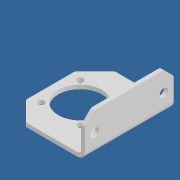
# Autodesk Inventor part: Belt_Unit_Motor_Holder
Saved by Autodesk Inventor 2020 (Build 240168000, 168)
## iProperties
Created: 2021-05-12
Part Number: Belt_Unit_Motor_Holder
Material: 一般
Document SubType Name: Sheet Metal
Designer: ken113
Density: 1 g/cm^3
Sheet Metal Rule: Default_mm
Appearance: 既定
Author: ken113
Autodesk Inventor part; units mm, degrees
ref_plane "YZ Plane" through (0, 0, 0) normal (1, 0, 0) x (0, 1, 0)
ref_plane "XZ Plane" through (0, 0, 0) normal (0, 1, 0) x (-1, 0, 0)
ref_plane "XY Plane" through (0, 0, 0) normal (0, 0, 1) x (1, 0, 0)
sketch "スケッチ1" plane through (0, 0, 0) normal (0, 1, 0) x (-1, 0, 0)
  line L0 (0, -22.5) -> (40, -22.5)
  line L1 (40, -22.5) -> (40, 22.5)
  line L2 (40, 22.5) -> (0, 22.5)
  line L3 (0, 22.5) -> (0, -22.5)
  point P0 (0, 0)
  dimension "d0" = 40
  dimension "d1" = 45
  dimension "d40" = 22.5
  measures "d0" distance of L1.end L2.end
  measures "d1" distance of L2.end L0.start
  measures "d40" distance from line of point (0, 0) L2
extrude "プレート1" add sketch "スケッチ1" along normal blind 2
sketch "スケッチ4" plane through (0, 2, 0) normal (0, 1, 0) x (1, 0, 0)
  circle A0 centre (-25, 0) radius 11.1
  line L0 (0, 22.5) -> (0, -22.5) projected
  point P0 (0, 0)
  dimension "d23" = 22.2
  dimension "d24" = 25
  constraints: 1 centre point
  measures "d23" diameter of A0
  measures "d24" distance from line of A0.centre L0
extrude "押し出し1" cut sketch "スケッチ4" against normal blind 10
sketch "スケッチ5" plane through (0, 2, 0) normal (0, 1, 0) x (1, 0, 0)
  circle A0 centre (-25, 0) radius 11.1 projected
  line L0 (0, 22.5) -> (0, -22.5) projected
  line L1 (-40, 22.5) -> (0, 22.5) projected
  line L2 (-40, -22.5) -> (-40, 22.5) projected
  line L3 (0, -22.5) -> (-40, -22.5) projected
  circle A1 centre (-25, 0) radius 14
  point P0 (0, 0)
  point P1 (-34.8995, -9.8995)
  point P2 (-15.1005, -9.8995)
  point P3 (-15.1005, 9.8995)
  point P4 (-34.8995, 9.8995)
  dimension "d28" = 28
  dimension "d31" = 360
  constraints: 1 coincident, 1 horizontal alignment, 8 other
hole "穴2" at (-34.8995, 2, 9.8995) at (-15.1005, 2, 9.8995) at (-15.1005, 2, -9.8995) at (-34.8995, 2, -9.8995) direction (0, -1, 0) diameter 3.2 end through all
sketch "スケッチ10" plane through (-2, 0, -22.5) normal (1, 0, 0) x (0, 1, 0)
  line L0 (0, 45) -> (0, 0)
  line L1 (0, 0) -> (20, 0)
  line L2 (20, 0) -> (20, 45)
  line L3 (20, 45) -> (0, 45)
  constraints: 6 end point, 1 horizontal, 1 perpendicular, 1 vertical
edge flange "フランジ4" height 20 angle 90 thickness 2 bend radius 2 thickness toward (1, 0, 0) relief straight relief width 2 relief depth 1 edges at (0, 2, 0) wall of the first edge with corners at (-2, 0, 22.5) (-2, 0, -22.5) (-2, 20, -22.5) (-2, 20, 22.5)
bend "曲げ4"
corner "コーナー4"
sketch "スケッチ12" plane through (-2, 20, -22.5) normal (-1, 0, 0) x (0, 0, 1)
  line L0 (0, -16) -> (45, -16) projected
  line L1 (45, -16) -> (45, 0) projected
  line L2 (45, 0) -> (0, 0) projected
  line L3 (0, -16) -> (0, 0) projected
  line L4 (40, -10) -> (5, -10)
  point P0 (22.5, -20)
  point P1 (22.5, -10)
  dimension "d77" = 35
  dimension "d78" = 10
  dimension "d79" = 22.5
  dimension "d80" = 45
  constraints: 2 end point, 1 horizontal, 1 horizontal alignment, 1 midpoint
  measures "d77" distance of L4.start L4.end
  measures "d78" distance from line of L2 L4.end
  measures "d79" distance from line of L3 point (22.5, -10)
  measures "d80" distance of L1.end L2.end
hole "穴3" at (-2, 10, -17.5) at (-2, 10, 17.5) direction (1, 0, 0) diameter 4.2 end through all
chamfer "面取り1" distance 10 angle 45 2 edges at (-40, 1, 22.5) (-40, 1, -22.5)
fillet "フィレット1" radius 2 4 edges at (-30, 1, -22.5) (-40, 1, -12.5) (-40, 1, 12.5) (-30, 1, 22.5)
chamfer "面取り2" distance 5 angle 45 2 edges at (-1, 20, 22.5) (-1, 20, -22.5)
fillet "フィレット2" radius 2 4 edges at (-1, 15, 22.5) (-1, 20, 17.5) (-1, 20, -17.5) (-1, 15, -22.5)
equation "\"d38\" = Thickness"
equation "\"d79\" = 0.5 * d80"
equation "\"d86\" = Thickness"
equation "\"d2\" = Thickness"
equation "\"d67\" = BendReliefWidth"
equation "\"d68\" = BendReliefDepth"
equation "\"d69\" = MinimumRemnant"
equation "\"d70\" = TransitionRadius"
equation "\"d73\" = BendRadius"
equation "\"d74\" = CornerReliefSize"
equation "\"d75\" = GapSize"
equation "\"d76\" = JacobiRadiusSize"
equation "\"d40\" = 0.5 * d1"
equation "\"BendRadius\" = Thickness"
equation "\"BendReliefWidth\" = Thickness"
equation "\"BendReliefDepth\" = 0.5 * Thickness"
equation "\"CornerReliefSize\" = 4 * Thickness"
equation "\"MinimumRemnant\" = 2 * Thickness"
equation "\"TransitionRadius\" = BendRadius"
equation "\"JacobiRadiusSize\" = BendRadius"
equation "\"GapSize\" = Thickness"
equation "\"Thickness\" = 2"
